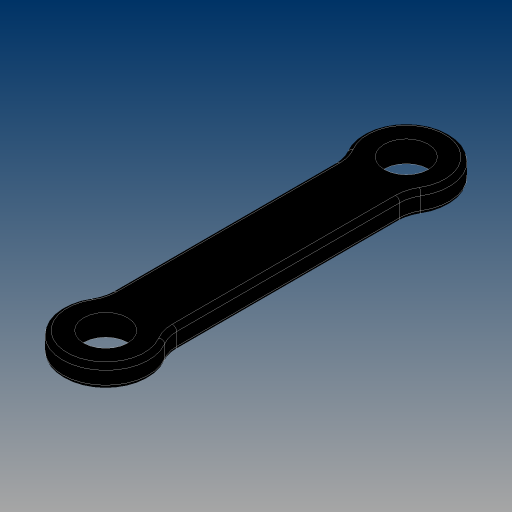
# Autodesk Inventor part: ELEV_044_CFSPRINGHOLDER
Saved by Autodesk Inventor 2024.3 (Build 283343000, 343)
## iProperties
Created: 2024-12-08
Part Number: ELEV_044_CFSPRINGHOLDER
Material: Aluminum 6061
Document SubType Name: Modeling
Designer: Kenji
Density: 2.7 g/cm^3
Appearance: Anodized - Black
Author: Kenji
Autodesk Inventor part; units mm, degrees
ref_plane "YZ Plane" through (0, 0, 0) normal (1, 0, 0) x (0, 1, 0)
ref_plane "XZ Plane" through (0, 0, 0) normal (0, 1, 0) x (-1, 0, 0)
ref_plane "XY Plane" through (0, 0, 0) normal (0, 0, 1) x (1, 0, 0)
sketch "Sketch1" plane through (0, 0, 0) normal (0, 1, 0) x (-1, 0, 0)
  circle A0 centre (0, 0) radius 3.2512
  circle A1 centre (0, -44.45) radius 3.2512
  circle A2 centre (0, 0) radius 6.35 construction
  circle A3 centre (0, -44.45) radius 6.35 construction
  line L0 (0, -6.35) -> (0, -38.1) construction
  line L1 (4.7625, -5.7238) -> (4.7625, -38.7262)
  line L2 (-4.7625, -5.7238) -> (-4.7625, -38.7262)
  arc A4 (5.4429, -3.2708) -> (-5.4429, -3.2708) centre (0, 0) ccw
  arc A5 (-5.4429, -41.1792) -> (5.4429, -41.1792) centre (0, -44.45) ccw
  arc A6 (5.4429, -3.2708) -> (4.7625, -5.7238) centre (9.525, -5.7238) ccw
  arc A7 (-4.7625, -5.7238) -> (-5.4429, -3.2708) centre (-9.525, -5.7238) ccw
  arc A8 (-5.4429, -41.1792) -> (-4.7625, -38.7262) centre (-9.525, -38.7262) ccw
  arc A9 (4.7625, -38.7262) -> (5.4429, -41.1792) centre (9.525, -38.7262) ccw
  point P0 (4.7625, -4.2001)
  point P1 (4.7625, -40.2499)
  point P2 (-4.7625, -4.2001)
  point P3 (-4.7625, -40.2499)
  dimension "d0" = 6.5024
  dimension "d1" = 44.45
  dimension "d2" = 12.7
  dimension "d3" = 4.7625
  dimension "d4" = 4.7625
  dimension "d5" = 4.7625
  constraints: 22 point on circle, 10 centre point, 8 tangent, 7 equal radius, 6 end point, 5 point on line, 3 coincident, 2 parallel, 1 concentric, 1 vertical, 1 vertical alignment
  measures "d0" diameter of A1
  measures "d1" distance of point (0, 0) A1.centre
  measures "d2" diameter of A3
  measures "d3" distance between parallel lines of L0 L1
  measures "d4" distance between parallel lines of L0 L2
  measures "d5" radius of A6
extrude "Extrusion1" add sketch "Sketch1" along normal blind 3.175
fillet "Fillet1" radius 0.635 16 edges at (-4.9357, 3.175, -4.451) (0, 3.175, 6.35) (4.9357, 3.175, -4.451) (4.7625, 3.175, -22.225) (4.9357, 3.175, -39.999) (0, 3.175, -50.8) (-4.9357, 3.175, -39.999) (-4.7625, 3.175, -22.225) (-4.9357, 0, -4.451) (0, 0, 6.35) (4.9357, 0, -4.451) (4.7625, 0, -22.225) (4.9357, 0, -39.999) (0, 0, -50.8) (-4.9357, 0, -39.999) (-4.7625, 0, -22.225)
body "Solid1"
